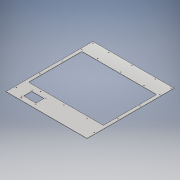
# Autodesk Inventor part: Front Cladding
Saved by Autodesk Inventor 2019 (Build 230136000, 136)
## iProperties
Created: 2018-10-13
Part Number: Front Cladding
Material: Aluminum 6061
Document SubType Name: Sheet Metal
Designer: Ax
Density: 2.7 g/cm^3
Sheet Metal Rule: Default_mm
Appearance: Anodized - Black
Mass: 496.154 g
Surface Area: 2509.97 cm^2
Volume: 183.761 cm^3
Flat Pattern Width: 51.3 cm
Flat Pattern Length: 55 cm
Flat Pattern Area: 2821.5 cm^2
Sheet Metal Width: 513.000 mm
Sheet Metal Length: 550.000 mm
Sheet Metal Area: 282150.000 mm^2
Author: Ax
Autodesk Inventor part; units mm, degrees
ref_plane "YZ Plane" through (0, 0, 0) normal (1, 0, 0) x (0, 1, 0)
ref_plane "XZ Plane" through (0, 0, 0) normal (0, 1, 0) x (-1, 0, 0)
ref_plane "XY Plane" through (0, 0, 0) normal (0, 0, 1) x (1, 0, 0)
sketch "Sketch1" plane through (0, 0, 0) normal (0, 0, 1) x (1, 0, 0)
  line L0 (-256.5, -275) -> (256.5, -275)
  line L1 (256.5, -275) -> (256.5, 275)
  line L2 (256.5, 275) -> (-256.5, 275)
  line L3 (-256.5, 275) -> (-256.5, -275)
  line L4 (-256.5, -275) -> (256.5, 275) construction
  line L5 (256.5, -275) -> (-256.5, 275) construction
  line L6 (-256.5, 265) -> (256.5, 265) construction
  line L7 (-246.5, 275) -> (-246.5, -275) construction
  line L8 (246.5, 275) -> (246.5, -275) construction
  line L9 (-256.5, -165) -> (256.5, -165) construction
  line L10 (-256.5, 195) -> (256.5, 195) construction
  circle A0 centre (-246.5, 265) radius 2.1
  circle A1 centre (-146.5, 265) radius 2.1
  circle A2 centre (146.5, 265) radius 2.1
  circle A3 centre (246.5, 265) radius 2.1
  circle A4 centre (146.5, 195) radius 2.1
  circle A5 centre (246.5, 195) radius 2.1
  circle A6 centre (-246.5, 195) radius 2.1
  circle A7 centre (-146.5, 195) radius 2.1
  line L11 (-146.5, 275) -> (-146.5, -275) construction
  line L12 (0, 0) -> (0, -275) construction
  line L13 (146.5, 275) -> (146.5, -275) construction
  circle A8 centre (-246.5, 70) radius 2.1
  circle A9 centre (146.5, -165) radius 2.1
  circle A10 centre (-146.5, -165) radius 2.1
  circle A11 centre (-246.5, -70) radius 2.1
  circle A12 centre (-246.5, -220) radius 2.1
  circle A13 centre (246.5, -220) radius 2.1
  circle A14 centre (246.5, -70) radius 2.1
  circle A15 centre (246.5, 70) radius 2.1
  line L14 (-246.5, 70) -> (246.5, 70) construction
  line L15 (-246.5, -70) -> (246.5, -70) construction
  line L16 (-246.5, 0) -> (246.5, 0) construction
  line L17 (-246.5, -220) -> (246.5, -220) construction
  line L18 (0, 275) -> (0, 0) construction
  circle A16 centre (0, 265) radius 2.1
  circle A17 centre (0, 195) radius 2.1
  circle A18 centre (0, -165) radius 2.1
  line L19 (-236.5, -152) -> (236.5, -152)
  line L20 (236.5, -152) -> (236.5, 185)
  line L21 (236.5, 185) -> (-236.5, 185)
  line L22 (-236.5, 185) -> (-236.5, -152)
  dimension "d0" = 513
  dimension "d1" = 550
  dimension "d2" = 10
  dimension "d3" = 10
  dimension "d4" = 10
  dimension "d5" = 110
  dimension "d6" = 80
  dimension "d7" = 110
  dimension "d8" = 110
  dimension "d9" = 70
  dimension "d10" = 55
  dimension "d11" = 4.2
  dimension "d14" = 10
  dimension "d15" = 10
  dimension "d17" = 13
  dimension "d18" = 10
  measures "d0" distance of L1.end L2.end
  measures "d1" distance of L0.end L1.end
  measures "d2" distance of L2.end L6.start
  measures "d3" distance of L0.start L7.end
  measures "d4" distance of L0.end L8.end
  measures "d5" distance of L0.end L9.end
  measures "d6" distance of L10.end L1.end
  measures "d7" distance of L0.start L11.end
  measures "d8" distance of L13.end L0.end
  measures "d9" vertical distance of L12.start L14.start
  measures "d10" vertical distance of L0.end L17.end
  measures "d11" diameter of A7
  measures "d14" distance between parallel lines of L10 L21
  measures "d15" distance between parallel lines of L8 L20
  measures "d17" distance from line of L9 L19.end
  measures "d18" distance between parallel lines of L7 L22
extrude "Plate4" add sketch "Sketch1" along normal blind 1.5
fillet "Fillet1" radius 5 4 edges at (-236.5, 185, 0.75) (236.5, 185, 0.75) (236.5, -152, 0.75) (-236.5, -152, 0.75)
sketch "Sketch2" plane through (0, 0, 1.5) normal (0, 0, 1) x (1, 0, 0)
  line L0 (-176.5, -192) -> (-98.05, -192)
  line L1 (-98.05, -192) -> (-98.05, -243)
  line L2 (-98.05, -243) -> (-176.5, -243)
  line L3 (-176.5, -243) -> (-176.5, -192)
  line L4 (256.5, 275) -> (256.5, -275) projected
  line L5 (231.5, -152) -> (-231.5, -152) projected
  line L6 (-256.5, -275) -> (-256.5, 275) projected
  point P0 (0, 0)
  dimension "d22" = 78.45
  dimension "d23" = 51
  dimension "d25" = 40
  dimension "d28" = 80
  constraints: 8 end point, 2 parallel, 1 horizontal, 1 perpendicular
  measures "d22" distance of L0.start L0.end
  measures "d23" distance of L0.end L1.end
  measures "d25" distance between parallel lines of L0 L5
  measures "d28" distance between parallel lines of L3 L6
extrude "Cut1" cut sketch "Sketch2" against normal blind 1.5
sketch "Sketch3" plane through (0, 0, 0) normal (0, 0, -1) x (-1, 0, 0)
  circle A0 centre (173.45, -261.3) radius 3.25
  line L0 (176.5, -243) -> (98.05, -243) projected
  point P0 (0, 0)
  dimension "d29" = 6.5
  dimension "d30" = 18.3
  dimension "d31" = 3.05
  constraints: 1 centre point
  measures "d29" diameter of A0
  measures "d30" distance from line of A0.centre L0
  measures "d31" horizontal distance of L0.start A0.centre
extrude "Cut2" cut sketch "Sketch3" against normal blind 1.5
sketch "Sketch4" plane through (0, 0, 0) normal (0, 0, -1) x (-1, 0, 0)
  line L0 (93.3, -250) -> (181.25, -250) construction
  line L1 (181.25, -250) -> (181.25, -185) construction
  line L2 (181.25, -185) -> (93.3, -185) construction
  line L3 (93.3, -185) -> (93.3, -250) construction
  line L4 (93.3, -250) -> (181.25, -185) construction
  line L5 (181.25, -250) -> (93.3, -185) construction
  line L6 (98.05, -243) -> (98.05, -192) construction
  line L7 (98.05, -217.5) -> (176.5, -217.5) construction
  line L8 (176.5, -192) -> (176.5, -243) construction
  circle A0 centre (181.25, -185) radius 1.7
  circle A1 centre (181.25, -250) radius 1.7
  circle A2 centre (93.3, -250) radius 1.7
  circle A3 centre (93.3, -185) radius 1.7
  point P0 (0, 0)
  point P1 (137.275, -217.5)
  point P2 (137.275, -217.5)
  dimension "d34" = 87.95
  dimension "d35" = 65
  dimension "d36" = 3.4
  constraints: 14 end point, 6 midpoint, 4 centre point, 4 coincident, 3 equal radius, 2 parallel, 2 perpendicular, 1 horizontal
  measures "d34" distance of L0.start L0.end
  measures "d35" distance of L2.end L0.start
  measures "d36" diameter of A0
hole "Hole1" at (-181.25, -250, 0) at (-181.25, -185, 0) at (-93.3, -185, 0) at (-93.3, -250, 0) direction (0, 0, 1) diameter 3.4 end through all
equation "\"d26\" = Thickness"
equation "\"d32\" = Thickness"
equation "\"d42\" = Thickness"
equation "\"d21\" = Thickness"
equation "\"BendRadius\" = Thickness"
equation "\"BendReliefWidth\" = Thickness"
equation "\"BendReliefDepth\" = 0.5 * Thickness"
equation "\"CornerReliefSize\" = 4 * Thickness"
equation "\"MinimumRemnant\" = 2 * Thickness"
equation "\"TransitionRadius\" = BendRadius"
equation "\"JacobiRadiusSize\" = BendRadius"
equation "\"GapSize\" = Thickness"
equation "\"d12\" = BendRadius"
equation "\"d13\" = BendRadius"
equation "\"d16\" = BendRadius"
equation "\"d19\" = BendRadius"
equation "\"Thickness\" = 1.5"
body "Solid4"
